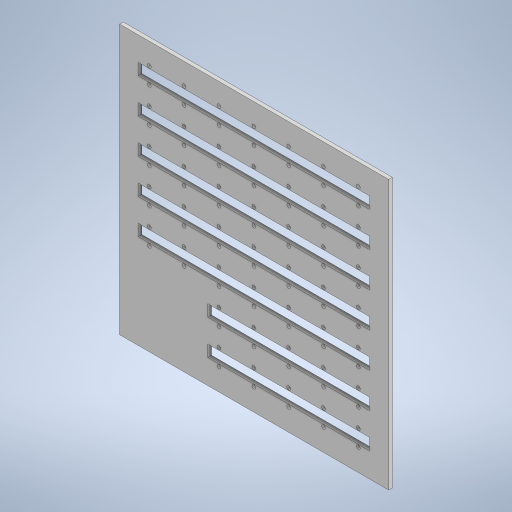
# Autodesk Inventor part: plade til motorer_MLH
Saved by Autodesk Inventor 2023 (Build 270158000, 158)
## iProperties
Created: 2022-06-14
Part Number: plade til motorer_MLH
Material: Generic
Document SubType Name: Modeling
Designer: Jakob Saugbjerg
Density: 1 g/cm^3
Appearance: Default
Author: Jakob Saugbjerg
Autodesk Inventor part; units mm, degrees
ref_plane "YZ Plane" through (0, 0, 0) normal (1, 0, 0) x (0, 1, 0)
ref_plane "XZ Plane" through (0, 0, 0) normal (0, 1, 0) x (-1, 0, 0)
ref_plane "XY Plane" through (0, 0, 0) normal (0, 0, 1) x (1, 0, 0)
sketch "Sketch1" plane through (0, 0, 0) normal (0, 0, 1) x (1, 0, 0)
  line L0 (0, 0) -> (220, 0)
  line L1 (220, 0) -> (220, 220)
  line L2 (220, 220) -> (0, 220)
  line L3 (0, 220) -> (0, 0)
  dimension "d0" = 220
  dimension "d1" = 220
  constraints: 8 end point, 2 parallel, 1 horizontal, 1 perpendicular
  measures "d0" distance of L2.end L1.end
  measures "d1" distance of L1.end L0.end
extrude "Extrusion1" add sketch "Sketch1" along normal blind 3
sketch "Sketch5" plane through (0, 0, 3) normal (0, 0, 1) x (1, 0, 0)
  circle A0 centre (24.25, 195.75) radius 10.25 projected
  circle A1 centre (24.25, 195.75) radius 10.25
  point P0 (0, 0)
  constraints: 1 centre point, 1 coincident
extrude "Extrusion5" add sketch "Sketch5" against normal blind 3
pattern_linear "Rectangular Pattern3" count 7 spacing 28.5 along (1, 0, 0) count 5 spacing 28.5 along (0, -1, 0) of "Extrusion5"
sketch "Sketch6" plane through (0, 0, 3) normal (0, 0, 1) x (1, 0, 0)
  circle A0 centre (195.25, 24.75) radius 10.25 projected
  circle A1 centre (195.25, 24.75) radius 10.25
  point P0 (0, 0)
  constraints: 1 centre point, 1 coincident
extrude "Extrusion6" add sketch "Sketch6" against normal blind 3
pattern_linear "Rectangular Pattern4" count 5 spacing 28.5 along (-1, 0, 0) count 2 spacing 28.5 along (0, 1, 0) of "Extrusion6"
sketch "Sketch7" plane through (195.25, 195.75, 0) normal (0, 0, -1) x (1, 0, 0)
  line L0 (0, 0) -> (0, -6.75)
  line L1 (0, -6.75) -> (0, 6.75)
  circle A0 centre (0, 6.75) radius 1.5
  circle A1 centre (0, -6.75) radius 1.5
  point P0 (-195.25, 195.75)
  dimension "d52" = 6.75
  dimension "d53" = 13.5
  dimension "d54" = 3
  dimension "d55" = 3
  constraints: 4 end point, 2 centre point, 2 coincident, 1 point on line, 1 vertical
  measures "d52" distance of L0.start L0.end
  measures "d53" distance of L0.end L1.end
  measures "d54" diameter of A0
  measures "d55" diameter of A1
extrude "Extrusion7" cut sketch "Sketch7" along normal mid plane 10
pattern_linear "Rectangular Pattern5" count 7 spacing 28.5 along (-1, 0, 0) count 5 spacing 28.5 along (0, -1, 0) of "Extrusion7"
sketch "Sketch8" plane through (195.25, 53.25, 0) normal (0, 0, -1) x (1, 0, 0)
  line L0 (0, 0) -> (0, -6.75)
  line L1 (0, -6.75) -> (0, 6.75)
  circle A0 centre (0, -6.75) radius 1.5
  circle A1 centre (0, 6.75) radius 1.5
  point P0 (-195.25, 53.25)
  dimension "d64" = 6.75
  dimension "d65" = 13.5
  dimension "d66" = 3
  dimension "d67" = 3
  constraints: 4 end point, 2 centre point, 2 coincident, 1 point on line, 1 vertical
  measures "d64" distance of L0.start L0.end
  measures "d65" distance of L0.end L1.end
  measures "d66" diameter of A0
  measures "d67" diameter of A1
extrude "Extrusion8" cut sketch "Sketch8" against normal blind 3
pattern_linear "Rectangular Pattern6" count 5 spacing 28.5 along (-1, 0, 0) count 2 spacing 28.5 along (0, -1, 0) of "Extrusion8"
sketch "Sketch9" plane through (195.25, 195.75, 0) normal (0, 0, -1) x (1, 0, 0)
  circle A0 centre (0, 0) radius 4.75
  line L0 (0, -4.75) -> (9.083, -4.75)
  circle A1 centre (0, 0) radius 10.25 projected
  circle A2 centre (-171, 0) radius 10.25 projected
  line L1 (9.083, -4.75) -> (-180.083, -4.75)
  line L2 (-180.083, -4.75) -> (-180.083, 4.75)
  line L3 (-180.083, 4.75) -> (9.083, 4.75)
  line L4 (9.083, 4.75) -> (9.083, -4.75)
  point P0 (-195.25, 195.75)
  dimension "d76" = 9.5
  constraints: 10 end point, 2 horizontal, 2 parallel, 1 perpendicular, 1 vertical alignment, 6 other
extrude "Extrusion9" cut sketch "Sketch9" against normal blind 3 contours A0
sketch "Sketch10" plane through (195.25, 195.75, 0) normal (0, 0, -1) x (1, 0, 0)
  circle A0 centre (0, 0) radius 4.75 projected
  line L0 (0, -4.75) -> (9.083, -4.75)
  circle A1 centre (0, 0) radius 10.25 projected
  circle A2 centre (-171, 0) radius 10.25 projected
  line L1 (9.083, -4.75) -> (-180.083, -4.75)
  line L2 (-180.083, -4.75) -> (-180.083, 4.75)
  line L3 (-180.083, 4.75) -> (9.083, 4.75)
  line L4 (9.083, 4.75) -> (9.083, -4.75)
  point P0 (-195.25, 195.75)
  point P1 (0, -4.75)
  constraints: 10 end point, 2 horizontal, 2 parallel, 1 perpendicular, 1 vertical alignment, 5 other
extrude "Extrusion10" cut sketch "Sketch10" against normal blind 6 contours A0 | L1 A1 L3 A0 | A0 L3 L4 L0 | L1 A2 L3 A1 | L1 L2 L3 A2
pattern_linear "Rectangular Pattern7" count 5 spacing 28.5 along (0, -1, 0) of "Extrusion10"
sketch "Sketch11" plane through (195.25, 53.25, 0) normal (0, 0, -1) x (1, 0, 0)
  circle A0 centre (0, 0) radius 4.75
  line L0 (0, -4.75) -> (9.083, -4.75)
  circle A1 centre (0, 0) radius 10.25 projected
  circle A2 centre (-114, 0) radius 10.25 projected
  line L1 (9.083, -4.75) -> (-123.083, -4.75)
  line L2 (-123.083, -4.75) -> (-123.083, 4.75)
  line L3 (-123.083, 4.75) -> (9.083, 4.75)
  line L4 (9.083, 4.75) -> (9.083, -4.75)
  point P0 (-195.25, 53.25)
  point P1 (-104.917, 4.75)
  point P2 (-104.917, -4.75)
  point P3 (0, -4.75)
  dimension "d84" = 9.5
  constraints: 10 end point, 2 horizontal, 2 parallel, 1 perpendicular, 1 vertical alignment, 6 other
extrude "Extrusion11" cut sketch "Sketch11" against normal blind 6 contours A0 | L1 A1 L3 A0 | A0 L3 L4 L0 | L1 A2 L3 A1 | L1 L2 L3 A2
pattern_linear "Rectangular Pattern9" count 2 spacing 28.5 along (0, -1, 0) of "Extrusion11"
body "Solid1"
